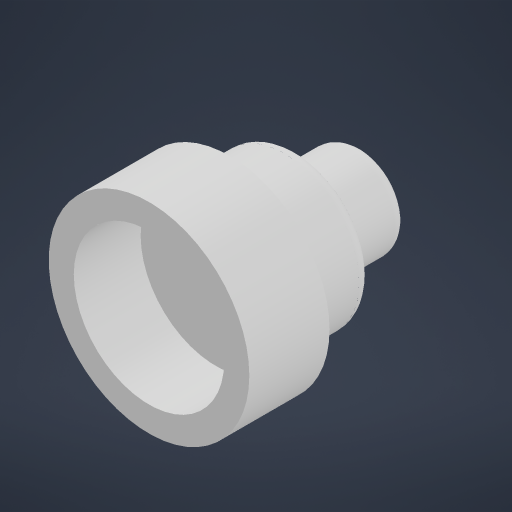
# Autodesk Inventor part: Elbow_Parallel_Rod_V1
Saved by Autodesk Inventor 2024.1 (Build 281209000, 209)
## iProperties
Created: 2023-06-29
Part Number: Elbow_Parallel_Rod_V1
Material: Generic
Document SubType Name: Modeling
Designer: User
Density: 1 g/cm^3
Appearance: Default
Author: User
Autodesk Inventor part; units mm, degrees
ref_plane "YZ Plane" through (0, 0, 0) normal (1, 0, 0) x (0, 1, 0)
ref_plane "XZ Plane" through (0, 0, 0) normal (0, 1, 0) x (-1, 0, 0)
ref_plane "XY Plane" through (0, 0, 0) normal (0, 0, 1) x (1, 0, 0)
sketch "Sketch1" plane through (0, 0, 0) normal (0, 0, 1) x (1, 0, 0)
  circle A0 centre (0, 0) radius 6.75
  dimension "d0" = 13.5
  constraints: 1 centre point, 1 coincident
  measures "d0" diameter of A0
extrude "Extrusion1" add sketch "Sketch1" along normal blind 15
sketch "Sketch2" plane through (0, 0, 15) normal (0, 0, 1) x (1, 0, 0)
  circle A0 centre (0, 0) radius 11.15
  circle A1 centre (0, 0) radius 12.75
  dimension "d3" = 22.3
  dimension "d19" = 25.5
  constraints: 2 centre point, 2 coincident
  measures "d3" diameter of A0
  measures "d19" diameter of A1
extrude "Extrusion3" add sketch "Sketch2" along normal blind 5 contours A0
sketch "Sketch3" plane through (0, 0, 15) normal (0, 0, -1) x (-1, 0, 0)
  circle A0 centre (0, 0) radius 10.15
  circle A1 centre (0, 0) radius 11.15
  dimension "d8" = 20.3
  dimension "d9" = 22.3
  constraints: 3 coincident, 2 centre point
  measures "d8" diameter of A0
  measures "d9" diameter of A1
extrude "Extrusion4" add sketch "Sketch3" along normal blind 5
sketch "Sketch4" plane through (0, 0, 20) normal (0, 0, 1) x (1, 0, 0)
  circle A0 centre (0, 0) radius 14.25
  dimension "d12" = 28.5
  constraints: 1 centre point, 1 coincident
  measures "d12" diameter of A0
extrude "Extrusion5" [suppressed]
fillet "Fillet1" [suppressed]
fillet "Fillet2" radius 2 1 edges at (-6.75, 0, 0)
fillet "Fillet3" radius 2 1 edges at (11.15, 0, 10)
fillet "Fillet4" [suppressed]
sketch "Sketch7" plane through (0, 0, 20) normal (0, 0, 1) x (1, 0, 0)
  circle A0 centre (0, 0) radius 15
  dimension "d20" = 30
  constraints: 1 centre point, 1 coincident
  measures "d20" diameter of A0
extrude "Extrusion6" add sketch "Sketch7" along normal blind 2
sketch "Sketch8" plane through (0, 0, 22) normal (0, 0, 1) x (1, 0, 0)
  circle A0 centre (0, 0) radius 11.25
  circle A1 centre (0, 0) radius 15
  dimension "d23" = 22.5
  dimension "d24" = 30
  constraints: 2 centre point, 2 coincident
  measures "d23" diameter of A0
  measures "d24" diameter of A1
extrude "Extrusion7" add sketch "Sketch8" along normal blind 10
body "Solid1"
